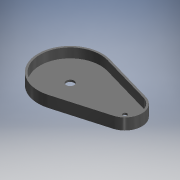
# Autodesk Inventor part: chain guard
Saved by Autodesk Inventor 2019 (Build 230136000, 136)
## iProperties
Part Number: chain guard
Material: Generic
Document SubType Name: Modeling
Designer: Delta
Appearance: Default
Author: Delta
Autodesk Inventor part; units mm, degrees
ref_plane "YZ Plane" through (0, 0, 0) normal (1, 0, 0) x (0, 1, 0)
ref_plane "XZ Plane" through (0, 0, 0) normal (0, 1, 0) x (-1, 0, 0)
ref_plane "XY Plane" through (0, 0, 0) normal (0, 0, 1) x (1, 0, 0)
sketch "Sketch1" plane through (0, 0, 0) normal (0, 1, 0) x (-1, 0, 0)
  circle A0 centre (0, 0) radius 53.975
  circle A1 centre (-92.202, 0) radius 28.575
  line L0 (-14.8691, 51.8865) -> (-100.0739, 27.4693)
  line L1 (-100.0739, -27.4693) -> (-14.8691, -51.8865)
  dimension "d0" = 107.95
  dimension "d1" = 57.15
  dimension "d2" = 92.202
  dimension "d3" = 0
  constraints: 4 end point, 4 point on circle, 4 tangent, 2 centre point, 1 coincident
  measures "d0" diameter of A0
  measures "d1" diameter of A1
  measures "d2" distance of A1.centre point (0, 0)
  measures "d3" vertical distance of point (0, 0) A1.centre
extrude "Extrusion1" add sketch "Sketch1" along normal blind 3.175
sketch "Sketch3" plane through (0, 3.175, 0) normal (0, 1, 0) x (1, 0, 0)
  point P0 (0, 0)
  point P1 (0, 0)
  constraints: 1 coincident
sketch "Sketch4" plane through (0, 3.175, 0) normal (0, 1, 0) x (1, 0, 0)
  arc A0 (100.0739, -27.4693) -> (100.0739, 27.4693) centre (92.202, 0) ccw projected
  point P0 (0, 0)
  constraints: 1 coincident
hole "Hole1" at (0, 3.175, 0) direction (0, -1, 0) diameter 13.208 end through all
hole "Hole2" at (92.202, 3.175, 0) direction (0, -1, 0) diameter 7.112 end through all
sketch "Sketch5" plane through (0, 3.175, 0) normal (0, 1, 0) x (1, 0, 0)
  circle A0 centre (0, 0) radius 50.8
  circle A1 centre (92.202, 0) radius 3.556 projected
  circle A2 centre (92.202, 0) radius 25.4
  line L0 (13.9945, -48.8344) -> (99.1992, -24.4172)
  line L1 (13.9945, 48.8344) -> (99.1992, 24.4172)
  line L2 (14.8691, -51.8865) -> (100.0739, -27.4693) projected
  arc A3 (14.8691, 51.8865) -> (14.8691, -51.8865) centre (0, 0) ccw projected
  line L3 (100.0739, 27.4693) -> (14.8691, 51.8865) projected
  arc A4 (100.0739, -27.4693) -> (100.0739, 27.4693) centre (92.202, 0) ccw projected
  dimension "d20" = 101.6
  dimension "d21" = 50.8
  constraints: 4 end point, 4 point on circle, 4 tangent, 2 centre point, 2 coincident
  measures "d20" diameter of A0
  measures "d21" diameter of A2
extrude "Extrusion2" add sketch "Sketch5" along normal blind 15.875 contours A3 L3 A4 L2
body "Solid1"
